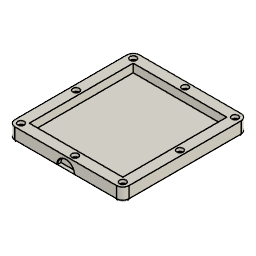
Case_Lid (Autodesk Fusion 360 design; units mm, degrees)
part number: 2026-03-28-22-40-39-091
Autodesk Fusion 360 part; units mm, degrees
sketch "Sketch1" plane through (0, 0, 0) normal (0, 0, 1) x (1, 0, 0)
  circle A0 centre (-43.1988, 54) radius 3.1
  arc A1 (-43.1988, 60) -> (-49.1988, 54) centre (-43.1988, 54) ccw
  circle A2 centre (55.8012, 0) radius 3.1
  line L0 (-49.1988, 54) -> (-49.1988, -54)
  circle A3 centre (-44.1988, 0) radius 3.1
  line L1 (50.8012, 50) -> (50.8012, -50)
  line L2 (50.8012, -50) -> (-39.1988, -50)
  circle A4 centre (9.8012, -55) radius 3.1
  line L3 (60.8012, -54) -> (60.8012, 54)
  circle A5 centre (54.8012, -54) radius 3.1
  line L4 (-43.1988, -60) -> (54.8012, -60)
  arc A6 (60.8012, 54) -> (54.8012, 60) centre (54.8012, 54) ccw
  line L5 (-39.1988, 50) -> (50.8012, 50)
  arc A7 (54.8012, -60) -> (60.8012, -54) centre (54.8012, -54) ccw
  circle A8 centre (-43.1988, -54) radius 3.1
  arc A9 (-49.1988, -54) -> (-43.1988, -60) centre (-43.1988, -54) ccw
  line L6 (-39.1988, -50) -> (-39.1988, 50)
  circle A10 centre (54.8012, 54) radius 3.1
  circle A11 centre (5.8012, 55) radius 3.1
  line L7 (54.8012, 60) -> (-43.1988, 60)
  dimension "d1" = 90
  dimension "d2" = 10
  dimension "d3" = 10
  dimension "d4" = 6.2
  dimension "d5" = 6.2
  dimension "d6" = 6.2
  dimension "d7" = 6
  dimension "d8" = 6
  dimension "d9" = 6
  dimension "d10" = 6
  dimension "d11" = 59
  dimension "d12" = 6.2
  dimension "d13" = 6.2
  dimension "d14" = 6
  dimension "d15" = 6
  dimension "d16" = 60
  dimension "d17" = 6.2
  dimension "d18" = 5
  dimension "d19" = 5
  dimension "d20" = 5
  dimension "d21" = 6.2
  dimension "d22" = 6
  dimension "d23" = 6
  dimension "d24" = 60
  dimension "d25" = 6.2
  dimension "d26" = 5
  dimension "d27" = 55
  dimension "d28" = 6
  dimension "d29" = 6
  dimension "d30" = 6
  dimension "d31" = 6
  constraint horizontal L5
  constraint vertical L1
  constraint horizontal L2
  constraint vertical L6
  constraint tangent L4 A9
  constraint tangent L0 A9
  constraint tangent L4 A7
  constraint tangent L3 A7
  constraint tangent L3 A6
  constraint tangent A6 L7
  constraint tangent A1 L0
  constraint tangent A1 L7
  measures "d1" distance of L1.start L5.start
  measures "d2" distance of L0 L6
  measures "d3" distance of L5 L7
  measures "d4" diameter of A4
  measures "d5" diameter of A5
  measures "d6" diameter of A8
  measures "d7" distance of A8.centre L0
  measures "d8" distance of A8.centre L4
  measures "d9" distance of A5.centre L3
  measures "d10" distance of A5.centre L4
  measures "d11" distance of A4.centre L0
  measures "d12" diameter of A2
  measures "d13" diameter of A10
  measures "d14" distance of A6.centre L7
  measures "d15" distance of A6.centre L3
  measures "d16" distance of A2.centre L7
  measures "d17" diameter of A3
  measures "d18" distance of A3.centre L0
  measures "d19" distance of A4.centre L2
  measures "d20" distance of A2.centre L3
  measures "d21" diameter of A0
  measures "d22" distance of A0.centre L0
  measures "d23" distance of A0.centre L7
  measures "d24" distance of A3.centre L4
  measures "d25" diameter of A11
  measures "d26" distance of A11.centre L7
  measures "d27" distance of A11.centre L3
  measures "d28" radius of A9
  measures "d29" radius of A7
  measures "d30" radius of A6
  measures "d31" radius of A1
extrude "Extrude1" add sketch "Sketch1" along normal blind 13
extrude "Extrude2" add sketch "Sketch1" along normal blind 5 contours L1 L2 L5 L6
extrude "Extrude3" add sketch "Sketch1" along normal blind 9.85 contours A0 | A2 | A3 | A4 | A5 | A8 | A10 | A11
sketch "Sketch2" plane through (0, -60, 0) normal (0, -1, 0) x (1, 0, 0)
  line L0 (-43.1988, 0) -> (54.8012, 0)
  line L1 (54.8012, 0) -> (54.8012, 13)
  line L2 (54.8012, 13) -> (-43.1988, 13)
  line L3 (-43.1988, 13) -> (-43.1988, 0)
  line L4 (5.8012, 2) -> (13.8012, 2)
  line L5 (5.8012, 2) -> (-2.1988, 2)
  arc A0 (13.8012, 2) -> (-2.1988, 2) centre (5.8012, 2) ccw
  dimension "d38" = 49
  dimension "d40" = 16
  dimension "d41" = 2
  constraint coincident L4.start L5.start
  constraint horizontal L4
  constraint parallel L4 L5
  measures "d38" distance of L1 L4.start
  measures "d40" diameter of A0
  measures "d41" distance of L0 L5
extrude "Extrude4" cut sketch "Sketch2" against normal blind 3.5 contours L4 L5 A0
sketch "Sketch3" plane through (0, -56.5, 0) normal (0, -1, 0) x (1, 0, 0)
  line L0 (7.0882, 9.85) -> (7.0882, 9.8958)
  arc A0 (7.0882, 9.8958) -> (-2.1988, 2) centre (5.8012, 2) ccw
  line L1 (-2.1988, 2) -> (13.8012, 2)
  arc A1 (13.8012, 2) -> (7.3431, 9.85) centre (5.8012, 2) ccw
  line L2 (7.3431, 9.85) -> (7.0882, 9.85)
fillet "Fillet1" radius 2 8 edges at (5.8012, 60, 0) (-47.4415, 58.2426, 0) (-49.1988, 0, 0) (-47.4415, -58.2426, 0) (5.8012, -60, 0) (59.0438, -58.2426, 0) (60.8012, 0, 0) (59.0438, 58.2426, 0)
fillet "Fillet2" radius 0.5 1 edges at (5.8012, -60, 10)
sketch "Sketch4" plane through (0, 0, 0) normal (0, 0, -1) x (1, 0, 0)
  line L0 (-43.1988, -58) -> (54.8012, -58)
  arc A0 (54.8012, -58) -> (58.8012, -54) centre (54.8012, -54) ccw
  line L1 (58.8012, -54) -> (58.8012, 54)
  arc A1 (58.8012, 54) -> (54.8012, 58) centre (54.8012, 54) ccw
  line L2 (54.8012, 58) -> (-43.1988, 58)
  arc A2 (-43.1988, 58) -> (-47.1988, 54) centre (-43.1988, 54) ccw
  line L3 (-47.1988, 54) -> (-47.1988, -54)
  arc A3 (-47.1988, -54) -> (-43.1988, -58) centre (-43.1988, -54) ccw
  line L4 (46.6066, -34.3989) -> (-34.9986, -34.378) construction
  line L5 (-34.9986, -34.378) -> (-35.0014, -45.622) construction
  line L6 (-35.0014, -45.622) -> (46.6038, -45.6429) construction
  line L7 (46.6038, -45.6429) -> (46.6066, -34.3989) construction
  dimension "d48" = 8
  dimension "d51" = 53
  text T0 "OMNAMOSIBIO" font "Arial" height 8 align centre middle in box 81.6052 x 11.2439 at (46.6066, -34.3989) x (-1, 0.000256) y (-0.000256, -1) spacing 1.005 kerned
extrude "Extrude5" cut sketch "Sketch4" against normal blind 4 text T0
sketch "Sketch5" plane through (0, 0, 0) normal (0, 0, 1) x (1, 0, 0)
  line L0 (51.8529, -22.4403) -> (-40.2506, 12.7155) construction
  line L1 (-40.2506, 12.7155) -> (-38.0253, 18.5453) construction
  line L2 (-38.0253, 18.5453) -> (54.0781, -16.6106) construction
  line L3 (54.0781, -16.6106) -> (51.8529, -22.4403) construction
  line L4 (58.8012, -54) -> (58.8012, 54)
  dimension "d54" = 9
  dimension "d56" = 53
  text T0 "PENDRIVE BOX" font "Arial" height 9 align centre middle in box 98.5848 x 6.24 at (51.8529, -22.4403) x (-0.934255, 0.356605) y (0.356605, 0.934255) spacing 1.005 kerned
extrude "Extrude6" cut sketch "Sketch5" along normal blind 4 text T0
equation "d49 = 'OMNAMOSIBIO'"
equation "d55 = 'PENDRIVE BOX'"
